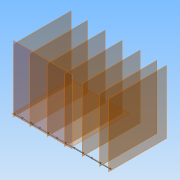
# Autodesk Inventor part: Pancake_Lever Shaft
Saved by Autodesk Inventor 2018.1 (Build 221171000, 171)
## iProperties
Created: 2019-02-22
Part Number: Pancake_Lever Shaft
Material: Stainless Steel
Document SubType Name: Modeling
Designer: James
Density: 8 g/cm^3
Appearance: Semi-Polished
Author: James
Autodesk Inventor part; units mm, degrees
ref_plane "YZ Plane" through (0, 0, 0) normal (1, 0, 0) x (0, 1, 0)
ref_plane "XZ Plane" through (0, 0, 0) normal (0, 1, 0) x (-1, 0, 0)
ref_plane "XY Plane" through (0, 0, 0) normal (0, 0, 1) x (1, 0, 0)
derived "Pancake_Skeleton.ipt"
ref_plane "Ground" through (0, 0, 0) normal (0, 1, 0) x (-1, 0, 0)
ref_plane "Back" through (0, 0, 0) normal (0, 0, 1) x (1, 0, 0)
ref_plane "LHS" through (0, 0, 0) normal (1, 0, 0) x (0, 1, 0)
ref_plane "Lane 1" through (90, 0, 0) normal (1, 0, 0) x (0, 1, 0)
ref_plane "Lane 2" through (185, 0, 0) normal (1, 0, 0) x (0, 1, 0)
ref_plane "Lane 3" through (280, 0, 0) normal (1, 0, 0) x (0, 1, 0)
ref_plane "Lane 4" through (375, 0, 0) normal (1, 0, 0) x (0, 1, 0)
ref_plane "Lane 5" through (470, 0, 0) normal (1, 0, 0) x (0, 1, 0)
ref_plane "RHS" through (520, 0, 0) normal (1, 0, 0) x (0, 1, 0)
sketch "Sketch2" plane through (0, 0, 0) normal (0, 0, 1) x (1, 0, 0)
  line L0 (0, 3.6) -> (0, -0.6) projected
  line L1 (90, 3.6) -> (90, -0.6) projected
  line L2 (185, 3.6) -> (185, -0.6) projected
  line L3 (280, 3.6) -> (280, -0.6) projected
  line L4 (375, 3.6) -> (375, -0.6) projected
  line L5 (470, 3.6) -> (470, -0.6) projected
  line L6 (520, 3.6) -> (520, -0.6) projected
  line L7 (-107, 0) -> (607, 0) projected
  line L8 (-5, 0) -> (525, 0)
  line L9 (525, 0) -> (525, 3)
  line L10 (525, 3) -> (-5, 3)
  line L11 (-5, 3) -> (-5, 0)
  line L12 (-107, 0) -> (607, 0) projected
  point P0 (0, 0)
  dimension "d3" = 3
  dimension "d22" = 5
  dimension "d23" = 5
  constraints: 8 end point, 2 parallel, 1 horizontal, 1 perpendicular, 1 point on line
  measures "d3" distance of L8.end L9.end
  measures "d22" distance between parallel lines of L0 L11
  measures "d23" distance between parallel lines of L6 L9
revolve "Revolution1" add sketch "Sketch2" angle 360 about axis through (-10, 0, 0) along (1, 0, 0)
sketch "Sketch3" plane through (0, 0, 0) normal (0, 0, 1) x (1, 0, 0)
  line L0 (41.5, 3) -> (42.3, 3)
  line L1 (42.3, 3) -> (42.3, 2.85)
  line L2 (42.3, 2.85) -> (41.5, 2.85)
  line L3 (41.5, 2.85) -> (41.5, 3)
  line L4 (-23.96, 0) -> (108.76, 0) projected
  line L5 (-5, -3) -> (-5, 3) projected
  line L6 (90, 4.2) -> (90, -4.2) projected
  line L7 (-23.96, 0) -> (108.76, 0) projected
  line L8 (37.2, 3) -> (38, 3)
  line L9 (38, 3) -> (38, 2.85)
  line L10 (38, 2.85) -> (37.2, 2.85)
  line L11 (37.2, 2.85) -> (37.2, 3)
  line L12 (185, 4.2) -> (185, -4.2) projected
  point P0 (0, 0)
  dimension "d5" = 0.8
  dimension "d6" = 2.85
  dimension "d20" = 0.8
  dimension "d21" = 3.5
  dimension "d31" = 95
  dimension "d32" = 48.5
  constraints: 16 end point, 4 parallel, 3 horizontal alignment, 2 horizontal, 2 perpendicular
  measures "d5" distance of L0.start L0.end
  measures "d6" distance between parallel lines of L4 L2
  measures "d20" distance of L8.start L8.end
  measures "d21" distance of L0.start L8.end
  measures "d31" distance between parallel lines of L12 L6
  measures "d32" distance from line of L6 L0.start
revolve "Revolution2" cut sketch "Sketch3" angle 360 about axis through (-10, 0, 0) along (1, 0, 0)
pattern_linear "Rectangular Pattern1" count 10 spacing 47.5 along (1, 0, 0) of "Revolution2"
sketch "Sketch4" plane through (0, 0, 0) normal (0, 0, 1) x (1, 0, 0)
  line L0 (15, 3) -> (15.8, 3)
  line L1 (15.8, 3) -> (15.8, 2.85)
  line L2 (15.8, 2.85) -> (15, 2.85)
  line L3 (15, 2.85) -> (15, 3)
  line L4 (-5, -3) -> (-5, 3) projected
  line L5 (-9.16, 0) -> (19.96, 0) projected
  line L6 (0, 4.2) -> (0, -4.2) projected
  line L7 (-9.16, 0) -> (19.96, 0) projected
  point P0 (0, 0)
  dimension "d14" = 2.85
  dimension "d15" = 0.8
  dimension "d17" = 15
  constraints: 8 end point, 2 parallel, 1 horizontal, 1 horizontal alignment, 1 perpendicular
  measures "d14" distance between parallel lines of L2 L5
  measures "d15" distance of L0.start L0.end
  measures "d17" distance from line of L0.start L6
revolve "Revolution3" [suppressed]
ref_plane "Mid Plane" through (260, 0, 0) normal (1, 0, 0) x (0, 1, 0)
mirror "Mirror1" [suppressed]
sketch "Sketch5" plane through (0, 0, 0) normal (0, 0, 1) x (1, 0, 0)
  line L0 (0, 4.2) -> (0, -4.2) projected
  line L1 (-22.94, 0) -> (102.64, 0) projected
  line L2 (-5, 3) -> (0, 3)
  line L3 (0, 3) -> (0, 1.5)
  line L4 (0, 1.5) -> (-5, 1.5)
  line L5 (-5, 1.5) -> (-5, 3)
  line L6 (37.2, 3) -> (37.2, -3) projected
  line L7 (-5, -3) -> (-5, 3) projected
  line L8 (-5, -3) -> (-5, 3) projected
  line L9 (-22.94, 0) -> (102.64, 0) projected
  point P0 (0, 0)
  dimension "d24" = 1.5
  dimension "d25" = 5
  constraints: 8 end point, 2 parallel, 1 coincident, 1 horizontal, 1 perpendicular, 1 point on line
  measures "d24" distance between parallel lines of L4 L1
  measures "d25" distance of L2.start L2.end
revolve "Revolution4" cut sketch "Sketch5" angle 360 about axis through (-10, 0, 0) along (1, 0, 0) contours L0 L4 L5 L2
mirror "Mirror2" about plane through (260, 0, 0) normal (1, 0, 0) of "Revolution4"
chamfer "Chamfer1" distance 0.5 angle 45 4 edges at (-5, -1.5, 0) (0, -3, 0) (525, -1.5, 0) (520, -3, 0)
fillet "Fillet1" radius 0.5 2 edges at (0, -1.5, 0) (520, -1.5, 0)
sketch "Sketch6" plane through (0, 0, 0) normal (0, 0, 1) x (1, 0, 0)
  line L0 (95.2, 3) -> (96, 3)
  line L1 (96, 3) -> (96, 2.85)
  line L2 (96, 2.85) -> (95.2, 2.85)
  line L3 (95.2, 2.85) -> (95.2, 3)
  line L4 (99.5, 3) -> (100.3, 3)
  line L5 (100.3, 3) -> (100.3, 2.85)
  line L6 (100.3, 2.85) -> (99.5, 2.85)
  line L7 (99.5, 2.85) -> (99.5, 3)
  line L8 (84.7, 3) -> (84.7, -3) projected
  line L9 (37.2, 3) -> (37.2, -3) projected
  line L10 (0.5, 3) -> (0.5, -3) projected
  line L11 (-111, 0) -> (631, 0) projected
  point P0 (0, 0)
  dimension "d36" = 10.5
  dimension "d37" = 0.8
  dimension "d38" = 0.8
  dimension "d39" = 3.5
  dimension "d40" = 2.85
  constraints: 16 end point, 4 parallel, 3 horizontal alignment, 2 horizontal, 2 perpendicular
  measures "d36" distance between parallel lines of L3 L8
  measures "d37" distance of L0.start L0.end
  measures "d38" distance of L4.start L4.end
  measures "d39" distance between parallel lines of L7 L1
  measures "d40" distance between parallel lines of L11 L2
revolve "Revolution5" cut sketch "Sketch6" angle 360 about axis through (-10, 0, 0) along (1, 0, 0)
equation "\"d20\" = d5"
equation "\"d38\" = d37"
body "Solid1"
